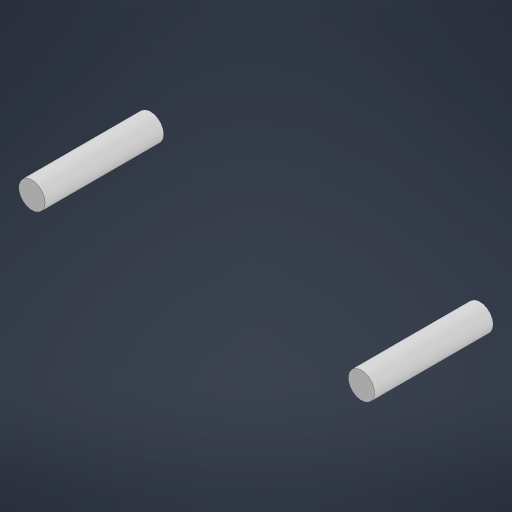
# Autodesk Inventor part: Topes_apm_002-2
Saved by Autodesk Inventor 2024 (Build 280153000, 153)
## iProperties
Created: 2023-05-13
Part Number: Topes_apm_002-2
Material: Genérico
Document SubType Name: Modeling
Designer: javie
Density: 1 g/cm^3
Appearance: Valor por defecto
Author: javie
Autodesk Inventor part; units mm, degrees
ref_plane "YZ Plane" through (0, 0, 0) normal (1, 0, 0) x (0, 1, 0)
ref_plane "XZ Plane" through (0, 0, 0) normal (0, 1, 0) x (-1, 0, 0)
ref_plane "Plano de trabajo1" through (-402.646, 112.0187, 0) normal (0, 0, 1) x (1, 0, 0)
sketch "Boceto1" plane through (-402.646, 112.0187, 0) normal (0, 0, 1) x (1, 0, 0)
  circle A0 centre (228.446, -104.9991) radius 2
  circle A1 centre (278.446, -104.9991) radius 2
  line L0 (-298.4, 16.0056) -> (-298.4, 11.0056)
  line L1 (0, 12.1063) -> (0, 7.1063)
  point P0 (402.646, -112.0187)
  dimension "d2" = 5
  dimension "d3" = 5
  dimension "d4" = 124.2
  dimension "d5" = 50
  constraints: 4 end point, 2 centre point, 2 vertical
  measures "d2" distance of L0.start L0.end
  measures "d3" distance of L1.start L1.end
  measures "d4" horizontal distance of point (402.646, -112.019) A1.centre
  measures "d5" distance of A1.centre A0.centre
extrude "Extrusión1" add sketch "Boceto1" along normal blind 18
